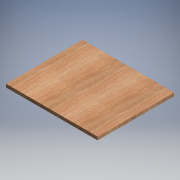
# Autodesk Inventor part: baseplate-mpx-bot
Saved by Autodesk Inventor 2016 (Build 200138000, 138)
## iProperties
Created: 2015-05-03
Part Number: baseplate-mpx-bot
Material: Wood (Birch)
Document SubType Name: Modeling
Designer: ax
Mass: 3465 g
Surface Area: 6462 cm^2
Volume: 6300 cm^3
Density: 0.55 g/cm^3
Appearance: Birch - Natural Polished
Author: ax
Autodesk Inventor part; units mm, degrees
ref_plane "YZ Plane" through (0, 0, 0) normal (1, 0, 0) x (0, 1, 0)
ref_plane "XZ Plane" through (0, 0, 0) normal (0, 1, 0) x (-1, 0, 0)
ref_plane "XY Plane" through (0, 0, 0) normal (0, 0, 1) x (1, 0, 0)
sketch "Sketch1" plane through (0, 0, 0) normal (0, 0, 1) x (1, 0, 0)
  line L0 (300, -250) -> (-300, -250)
  line L1 (-300, -250) -> (-300, 250)
  line L2 (-300, 250) -> (300, 250)
  line L3 (300, 250) -> (300, -250)
  line L4 (300, -250) -> (-300, 250) construction
  line L5 (-300, -250) -> (300, 250) construction
  point P0 (0, 0)
  dimension "d0" = 600
  dimension "d1" = 500
  constraints: 12 end point, 2 midpoint, 2 parallel, 1 horizontal, 1 perpendicular
  measures "d0" distance of L1.end L2.end
  measures "d1" distance of L0.end L1.end
extrude "Extrusion1" add sketch "Sketch1" along normal blind 21
body "Solid1"
